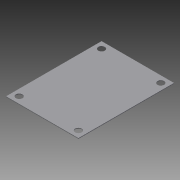
# Autodesk Inventor part: mainPCB
Saved by Autodesk Inventor 2015 (Build 190159000, 159)
## iProperties
Created: 2015-02-12
Part Number: mainPCB
Material: Generic
Document SubType Name: Modeling
Designer: 477grp12
Density: 1 g/cm^3
Appearance: Default
Mass: 1.97753 g
Surface Area: 79.4676 cm^2
Volume: 1.97753 cm^3
Author: 477grp12
Autodesk Inventor part; units mm, degrees
ref_plane "YZ Plane" through (0, 0, 0) normal (1, 0, 0) x (0, 1, 0)
ref_plane "XZ Plane" through (0, 0, 0) normal (0, 1, 0) x (-1, 0, 0)
ref_plane "XY Plane" through (0, 0, 0) normal (0, 0, 1) x (1, 0, 0)
sketch "Sketch1" plane through (0, 0, 0) normal (0, 1, 0) x (-1, 0, 0)
  line L0 (0, 0) -> (54.86, 0)
  line L1 (54.86, 0) -> (54.86, -72.39)
  line L2 (54.86, -72.39) -> (0, -72.39)
  line L3 (0, -72.39) -> (0, 0)
  dimension "d0" = 54.86
  dimension "d1" = 72.39
  constraints: 8 end point, 2 parallel, 1 horizontal, 1 perpendicular
  measures "d0" distance of L1.end L2.end
  measures "d1" distance of L2.end L0.start
extrude "Extrusion1" add sketch "Sketch1" along normal blind 0.508
sketch "Sketch2" plane through (0, 0.508, 0) normal (0, 1, 0) x (1, 0, 0)
  line L0 (-33.1258, 25.0435) -> (-33.1258, 49.6219) construction
  line L1 (-33.1258, 49.6219) -> (-23.1073, 49.6219) construction
  line L2 (-23.1073, 49.6219) -> (-23.1073, 25.0435) construction
  line L3 (-23.1073, 25.0435) -> (-33.1258, 25.0435) construction
  circle A0 centre (-49.86, 5) radius 1.5
  circle A1 centre (-49.86, 67.39) radius 1.5
  circle A2 centre (-5, 5) radius 1.5
  circle A3 centre (-5, 67.39) radius 1.5
  line L4 (-54.86, 72.39) -> (0, 72.39) projected
  line L5 (-54.86, 0) -> (-54.86, 72.39) projected
  line L6 (0, 0) -> (0, 72.39) projected
  line L7 (0, 0) -> (-54.86, 0) projected
  dimension "d4" = 3
  dimension "d5" = 3
  dimension "d6" = 3
  dimension "d7" = 3
  dimension "d15" = 5
  dimension "d16" = 5
  dimension "d17" = 5
  dimension "d18" = 5
  constraints: 4 centre point, 2 other
  measures "d4" diameter of A0
  measures "d5" diameter of A1
  measures "d6" diameter of A2
  measures "d7" diameter of A3
  measures "d15" distance from line of L4 A1.centre
  measures "d16" distance from line of L5 A1.centre
  measures "d17" distance from line of L6 A2.centre
  measures "d18" distance from line of L7 A2.centre
hole "Hole1" at (-49.86, 0.508, -67.39) at (-49.86, 0.508, -5) at (-5, 0.508, -5) at (-5, 0.508, -67.39) direction (0, -1, 0) diameter 5 end through all
body "Solid1"
